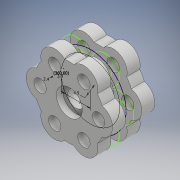
# Autodesk Inventor part: piston-star-connector
Saved by Autodesk Inventor 2018 (Build 220112000, 112)
## iProperties
Created: 2025-02-25
Part Number: piston-star-connector
Material: Generic
Document SubType Name: Modeling
Designer: neo
Density: 1 g/cm^3
Appearance: Default
Author: neo
Autodesk Inventor part; units mm, degrees
ref_plane "YZ Plane" through (0, 0, 0) normal (1, 0, 0) x (0, 1, 0)
ref_plane "XZ Plane" through (0, 0, 0) normal (0, 1, 0) x (-1, 0, 0)
ref_plane "XY Plane" through (0, 0, 0) normal (0, 0, 1) x (1, 0, 0)
sketch "Sketch1" plane through (0, 0, 0) normal (0, 1, 0) x (-1, 0, 0)
  circle A0 centre (9, 0) radius 1.9
  circle A1 centre (4.5, 7.7942) radius 1.9
  circle A2 centre (-4.5, 7.7942) radius 1.9
  circle A3 centre (-9, 0) radius 1.9
  circle A4 centre (-4.5, -7.7942) radius 1.9
  circle A5 centre (4.5, -7.7942) radius 1.9
  circle A6 centre (9, 0) radius 4.3
  circle A7 centre (4.5, 7.7942) radius 4.3
  circle A8 centre (-4.5, 7.7942) radius 4.3
  circle A9 centre (-9, 0) radius 4.3
  circle A10 centre (-4.5, -7.7942) radius 4.3
  circle A11 centre (4.5, -7.7942) radius 4.3
  circle A12 centre (0, 0) radius 10.9
  circle A13 centre (0, 0) radius 2.25
  circle A14 centre (0, 0) radius 4.7
  dimension "d0" = 3.8
  dimension "d1" = 9
  dimension "d4" = 360
  dimension "d6" = 2.4
  dimension "d9" = 360
  dimension "d13" = 4.5
  constraints: 15 centre point, 5 coincident, 2 tangent, 26 other
  measures "d0" diameter of A0
  measures "d1" distance of point (0, 0) A0.centre
  measures "d6" radial gap between concentric circles of A0 A6
  measures "d13" diameter of A13
extrude "Extrusion1" add sketch "Sketch1" along normal mid plane 13 contours A12 A6 | A12 A6 | A6 A14 A7 A12 | A12 A11 A14 A6 | A14 | A12 A7 | A7 A12 | A12 A11 | A11 A12 | A14 A8 A12 A7 | A11 A12 A10 A14 | A14 A9 A12 A8 | A8 A12 | A10 A12 | A10 A12 A9 A14 | A12 A8 | A9 A12 | A10 A12 | A12 A9 | A13
extrude "Extrusion2" cut sketch "Sketch1" along normal through all both and the other way through all contours A13
extrude "Extrusion3" cut sketch "Sketch1" along normal mid plane 5
extrude "Extrusion4" add sketch "Sketch1" along normal through all both and the other way through all contours A14
hole "Hole1" at (0, 6.5, 0) direction (0, -1, 0) diameter 5 end through all counterbore diameter 8 counterbore depth 2
mirror "Mirror1" about plane through (0, 0, 0) normal (0, 1, 0) of "Hole1"
body "Solid1"
